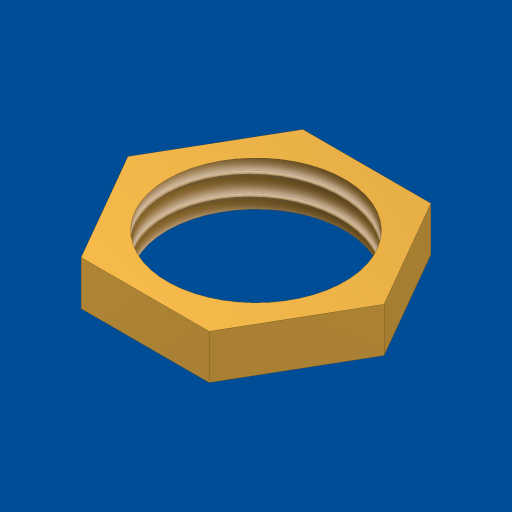
# Autodesk Inventor part: rp-sma_nut
Saved by Autodesk Inventor 2023.2 (Build 272271000, 271)
## iProperties
Created: 2023-01-27
Part Number: rp-sma_nut
Material: Brass, Soft Yellow
Document SubType Name: Modeling
Designer: agmlego
Mass: 0.307832 g
Surface Area: 1.21107 cm^2
Volume: 0.0363439 cm^3
Density: 8.47 g/cm^3
Appearance: Brass - Satin
Author: agmlego
Autodesk Inventor part; units mm, degrees
ref_plane "YZ Plane" through (0, 0, 0) normal (1, 0, 0) x (0, 1, 0)
ref_plane "XZ Plane" through (0, 0, 0) normal (0, 1, 0) x (-1, 0, 0)
ref_plane "XY Plane" through (0, 0, 0) normal (0, 0, 1) x (1, 0, 0)
sketch "Sketch1" plane through (0, 0, 0) normal (0, 1, 0) x (-1, 0, 0)
  line L0 (4.5827, 0) -> (2.2914, -3.9688)
  line L1 (2.2914, -3.9688) -> (-2.2914, -3.9687)
  line L2 (-2.2914, -3.9687) -> (-4.5827, 0)
  line L3 (-4.5827, 0) -> (-2.2914, 3.9688)
  line L4 (-2.2914, 3.9688) -> (2.2914, 3.9688)
  line L5 (2.2914, 3.9688) -> (4.5827, 0)
  circle A0 centre (0, 0) radius 3.175
  dimension "d0" = 7.9375
  dimension "d1" = 6.35
  constraints: 12 end point, 2 coincident, 1 centre point, 13 other
  measures "d0" distance between parallel lines of L1 L4
  measures "d1" diameter of A0
extrude "Extrusion1" add sketch "Sketch1" along normal blind 1.5875
thread "Thread1" size "1/4-36 UNS" class "2B" standard "ANSI Unified Screw Threads" full length
body "Solid1"
